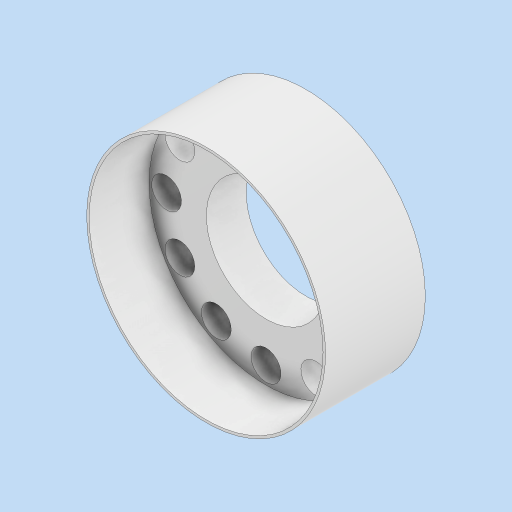
# Autodesk Inventor part: HubCap_v7
Saved by Autodesk Inventor 2023 (Build 270158000, 158)
## iProperties
Created: 2023-04-06
Part Number: HubCap_v7
Material: ABS Plastic
Document SubType Name: Modeling
Designer: asach
Density: 1.06 g/cm^3
Appearance: Smooth - White
Author: asach
Autodesk Inventor part; units mm, degrees
ref_plane "YZ Plane" through (0, 0, 0) normal (1, 0, 0) x (0, 1, 0)
ref_plane "XZ Plane" through (0, 0, 0) normal (0, 1, 0) x (-1, 0, 0)
ref_plane "XY Plane" through (0, 0, 0) normal (0, 0, 1) x (1, 0, 0)
sketch "Sketch1" plane through (0, 0, 0) normal (0, 0, 1) x (1, 0, 0)
  circle A0 centre (0, 0) radius 38.1
  circle A1 centre (0, 0) radius 37.3
  circle A2 centre (0, 0) radius 19.05
  circle A3 centre (0, 0) radius 31.75 construction
  circle A4 centre (0, -31.75) radius 4.7625
  line L0 (0, -53.34) -> (0, 53.34) construction
  dimension "d7" = 63.5
  dimension "d0" = 76.2
  dimension "d1" = 0.8
  dimension "d4" = 38.1
  dimension "d8" = 9.525
  constraints: 4 centre point, 3 coincident, 1 point on line, 1 vertical alignment, 2 other
  measures "d0" diameter of A0
  measures "d1" radial gap between concentric circles of A0 A1
  measures "d4" diameter of A2
  measures "d8" diameter of A4
extrude "Extrusion1" add sketch "Sketch1" along normal blind 31.825 contours A0
extrude "Extrusion2" add sketch "Sketch1" along normal blind 12.7 contours A1 | A4
extrude "Extrusion3" cut sketch "Sketch1" along normal through all contours A4
pattern_circular "Circular Pattern1" count 12 over 360 about axis through (0, 0, 0) along (0, 0, 1) of "Extrusion3"
body "Solid1"
